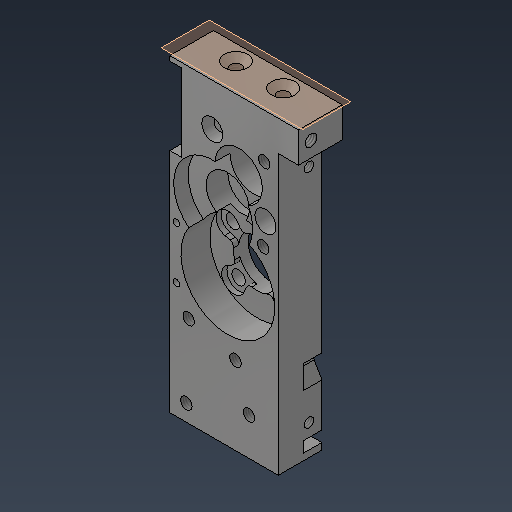
# Autodesk Inventor part: RightGearbox
Saved by Autodesk Inventor 2026.2 (Build 302298010, 298A)
## iProperties
Created: 2026-04-14
Part Number: RightGearbox
Material: Steel
Document SubType Name: Sheet Metal
Designer: szymo
Density: 7.85 g/cm^3
Appearance: Nylon 6(1)
Mass: 69.272 g
Surface Area: 68.2976 cm^2
Volume: 8.82446 cm^3
Sheet Metal Rule: Default
Author: szymo
Autodesk Inventor part; units mm, degrees
(part 1 of 2)
ref_plane "YZ Plane" through (0, 0, 0) normal (1, 0, 0) x (0, 1, 0)
ref_plane "XZ Plane" through (0, 0, 0) normal (0, 1, 0) x (-1, 0, 0)
ref_plane "XY Plane" through (0, 0, 0) normal (0, 0, 1) x (1, 0, 0)
sketch "Sketch1" plane through (0, 0, 0) normal (0, 0, 1) x (1, 0, 0)
  circle A0 centre (14.7, -14.7) radius 5
  circle A1 centre (14.7, -14.7) radius 14.7 construction
  circle A2 centre (14.7, -55.637072) radius 5
  circle A3 centre (14.7, -55.637072) radius 14.7 construction
  line L0 (23.1, 0) -> (0, 0)
  line L1 (0, 0) -> (0, -65.837072)
  line L2 (0, -65.837072) -> (23.1, -65.837072)
  line L3 (23.1, -65.837072) -> (23.1, 0)
  circle A4 centre (12.35, -35.272213) radius 5
  line L4 (23.43749, -53.479232) -> (27.439125, -51.168886)
  arc A5 (27.439125, -51.168886) -> (24.939125, -46.838759) centre (14.7, -55.637072) ccw
  line L5 (24.939125, -46.838759) -> (20.93749, -49.149105)
  arc A6 (23.43749, -53.479232) -> (20.93749, -49.149105) centre (14.7, -55.637072) ccw construction
  arc A7 (1.960875, -60.105258) -> (4.460875, -64.435385) centre (14.7, -55.637072) ccw
  line L6 (1.960875, -60.105258) -> (5.96251, -57.794913)
  line L7 (8.46251, -62.12504) -> (4.460875, -64.435385)
  line L8 (23.43749, -53.479232) -> (23.1, -53.479232)
  line L9 (24.939125, -46.838759) -> (23.1, -46.838759)
  line L10 (8.46251, -62.12504) -> (5.96251, -57.794913)
  line L11 (23.43749, -53.479232) -> (20.93749, -49.149105)
  line L12 (8.46251, -62.12504) -> (23.1, -62.12504)
  circle A8 centre (9.222618, -23.066498) radius 4.2 construction
  circle A9 centre (9.222618, -23.066498) radius 8 construction
  circle A10 centre (12.35, -35.272213) radius 9.6 construction
  circle A11 centre (12.35, -35.272213) radius 10
  circle A12 centre (9.222618, -23.066498) radius 4.6
  circle A13 centre (9.222618, -23.066498) radius 8.4
  arc A14 (5.96251, -57.794913) -> (8.46251, -62.12504) centre (14.7, -55.637072) ccw construction
  line L13 (2.5, -1) -> (1.5, -1)
  line L14 (1.5, -1) -> (1.5, -17)
  line L15 (1.5, -17) -> (2.5, -17)
  line L16 (2.5, -17) -> (2.5, -1)
  line L17 (1.5, -1) -> (1, -1)
  line L18 (1, -1) -> (1, -1)
  line L19 (1, -1) -> (0, -1)
  line L20 (2.5, -17) -> (2.5, -17.5)
  line L21 (2.5, -17.5) -> (1, -17.5)
  line L22 (1, -17.5) -> (1, -17.5)
  line L23 (1, -17.5) -> (0, -17.5)
  line L24 (23.1, 0) -> (27.4, 0)
  line L25 (27.4, 0) -> (27.4, -6.5)
  line L26 (27.4, -6.5) -> (23.1, -6.5)
  line L27 (24.939125, -23.498313) -> (20.93749, -21.187968)
  arc A15 (20.93749, -21.187968) -> (23.43749, -16.857841) centre (14.7, -14.7) ccw
  line L28 (23.43749, -16.857841) -> (27.439125, -19.168186)
  arc A16 (24.939125, -23.498313) -> (27.439125, -19.168186) centre (14.7, -14.7) ccw
  circle A17 centre (14.7, -14.7) radius 14.7 construction
  circle A18 centre (14.7, -14.7) radius 14 construction
  circle A19 centre (14.7, -14.7) radius 5
  circle A20 centre (14.7, -14.7) radius 14 construction
  line L29 (22.512272, -20.942468) -> (24.697093, -22.203875) construction
  arc A21 (22.512272, -20.942468) -> (24.012272, -18.344392) centre (14.7, -14.7) ccw construction
  line L30 (26.197093, -19.605799) -> (24.012272, -18.344392) construction
  arc A22 (24.697093, -22.203875) -> (26.197093, -19.605799) centre (14.7, -14.7) ccw construction
  circle A23 centre (14.7, -55.637072) radius 14.7 construction
  circle A24 centre (14.7, -55.637072) radius 14 construction
  line L31 (22.512272, -49.394604) -> (24.697093, -48.133197)
  arc A25 (26.197093, -50.731273) -> (24.697093, -48.133197) centre (14.7, -55.637072) ccw
  line L32 (26.197093, -50.731273) -> (24.012272, -51.99268)
  arc A26 (24.012272, -51.99268) -> (22.512272, -49.394604) centre (14.7, -55.637072) ccw
  arc A27 (3.202907, -60.542871) -> (4.702907, -63.140947) centre (14.7, -55.637072) ccw
  line L33 (3.202907, -60.542871) -> (5.387728, -59.281464)
  arc A28 (5.387728, -59.281464) -> (6.887728, -61.87954) centre (14.7, -55.637072) ccw
  line L34 (6.887728, -61.87954) -> (4.702907, -63.140947)
  circle A29 centre (14.7, -55.637072) radius 5
  circle A30 centre (14.7, -55.637072) radius 14 construction
  arc A31 (15.739868, -27.750823) -> (15.831115, -26.325602) centre (9.837244, -26.657388) ccw
  arc A32 (15.831115, -26.325602) -> (15.358114, -26.155676) centre (12.35, -35.272213) ccw
  arc A33 (15.358114, -26.155676) -> (14.521528, -27.313132) centre (19.770536, -30.225947) ccw
  arc A34 (14.521528, -27.313132) -> (14.102006, -27.210391) centre (12.35, -35.272213) ccw
  arc A35 (14.102006, -27.210391) -> (13.894939, -25.797343) centre (8.101031, -27.368074) ccw
  arc A36 (13.894939, -25.797343) -> (13.396945, -25.729472) centre (12.35, -35.272213) ccw
  arc A37 (13.396945, -25.729472) -> (12.819289, -27.035571) centre (18.559202, -28.793404) ccw
  arc A38 (12.819289, -27.035571) -> (12.387574, -27.022298) centre (12.35, -35.272213) ccw
  arc A39 (12.387574, -27.022298) -> (11.891242, -25.68318) centre (6.550518, -28.424209) ccw
  arc A40 (11.891242, -25.68318) -> (11.39002, -25.720331) centre (12.35, -35.272213) ccw
  arc A41 (11.39002, -25.720331) -> (11.09654, -27.117991) centre (17.076495, -27.644016) ccw
  arc A42 (11.09654, -27.117991) -> (10.671499, -27.194767) centre (12.35, -35.272213) ccw
  arc A43 (10.671499, -27.194767) -> (9.907595, -25.988105) centre (5.253471, -29.779634) ccw
  arc A44 (9.907595, -25.988105) -> (9.42505, -26.128654) centre (12.35, -35.272213) ccw
  arc A45 (9.42505, -26.128654) -> (9.428573, -27.556789) centre (15.387219, -26.828017) ccw
  arc A46 (9.428573, -27.556789) -> (9.028783, -27.720258) centre (12.35, -35.272213) ccw
  arc A47 (9.028783, -27.720258) -> (8.030693, -26.698789) centre (4.266575, -31.375112) ccw
  arc A48 (8.030693, -26.698789) -> (7.587914, -26.936594) centre (12.35, -35.272213) ccw
  arc A49 (7.587914, -26.936594) -> (7.888286, -28.332788) centre (13.565201, -26.381069) ccw
  arc A50 (7.888286, -28.332788) -> (7.53122, -28.575807) centre (12.35, -35.272213) ccw
  arc A51 (7.53122, -28.575807) -> (6.342565, -27.784174) centre (3.632965, -33.140911) ccw
  arc A52 (6.342565, -27.784174) -> (5.958905, -28.108841) centre (12.35, -35.272213) ccw
  arc A53 (5.958905, -28.108841) -> (6.542998, -29.412074) centre (11.690074, -26.322707) ccw
  arc A54 (6.542998, -29.412074) -> (6.24426, -29.72402) centre (12.35, -35.272213) ccw
  arc A55 (6.24426, -29.72402) -> (4.916991, -29.196821) centre (3.380331, -34.999859) ccw
  arc A56 (4.916991, -29.196821) -> (4.609216, -29.594161) centre (12.35, -35.272213) ccw
  arc A57 (4.609216, -29.594161) -> (5.451504, -30.747475) centre (9.843788, -26.655482) ccw
  arc A58 (5.451504, -30.747475) -> (5.224151, -31.114716) centre (12.35, -35.272213) ccw
  arc A59 (5.224151, -31.114716) -> (3.816275, -30.874993) centre (3.519714, -36.87071) ccw
  arc A60 (3.816275, -30.874993) -> (3.597838, -31.327639) centre (12.35, -35.272213) ccw
  arc A61 (3.597838, -31.327639) -> (4.661507, -32.28063) centre (8.107035, -27.364849) ccw
  arc A62 (4.661507, -32.28063) -> (4.515476, -32.687114) centre (12.35, -35.272213) ccw
  arc A63 (4.515476, -32.687114) -> (3.088524, -32.745344) centre (4.045023, -38.671698) ccw
  arc A64 (3.088524, -32.745344) -> (2.968971, -33.233515) centre (12.35, -35.272213) ccw
  arc A65 (2.968971, -33.233515) -> (4.207533, -33.944531) centre (6.555721, -28.419806) ccw
  arc A66 (4.207533, -33.944531) -> (4.149207, -34.372494) centre (12.35, -35.272213) ccw
  arc A67 (4.149207, -34.372494) -> (2.765544, -34.726131) centre (4.933299, -40.324113) ccw
  arc A68 (2.765544, -34.726131) -> (2.7501, -35.228491) centre (12.35, -35.272213) ccw
  arc A69 (2.7501, -35.228491) -> (4.109425, -35.666458) centre (5.257644, -29.774246) ccw
  arc A70 (4.109425, -35.666458) -> (4.141352, -36.097196) centre (12.35, -35.272213) ccw
  arc A71 (4.141352, -36.097196) -> (2.861451, -36.730784) centre (6.145721, -41.755736) ccw
  arc A72 (2.861451, -36.730784) -> (2.95079, -37.225378) centre (12.35, -35.272213) ccw
  arc A73 (2.95079, -37.225378) -> (4.37147, -37.371154) centre (4.269538, -31.368973) ccw
  arc A74 (4.37147, -37.371154) -> (4.492254, -37.785842) centre (12.35, -35.272213) ccw
  arc A75 (4.492254, -37.785842) -> (3.372052, -38.671691) centre (7.6293, -42.903997) ccw
  arc A76 (3.372052, -38.671691) -> (3.562271, -39.136902) centre (12.35, -35.272213) ccw
  arc A77 (3.562271, -39.136902) -> (4.982214, -38.984117) centre (3.634586, -33.134291) ccw
  arc A78 (4.982214, -38.984117) -> (5.186578, -39.36463) centre (12.35, -35.272213) ccw
  arc A79 (5.186578, -39.36463) -> (4.275033, -40.464025) centre (9.319196, -43.718713) ccw
  arc A80 (4.275033, -40.464025) -> (4.557818, -40.879521) centre (12.35, -35.272213) ccw
  arc A81 (4.557818, -40.879521) -> (5.914967, -40.434852) centre (3.38054, -34.993046) ccw
  arc A82 (5.914967, -40.434852) -> (6.193977, -40.76456) centre (12.35, -35.272213) ccw
  arc A83 (6.193977, -40.76456) -> (5.530929, -42.029451) centre (11.141552, -44.164277) ccw
  arc A84 (5.530929, -42.029451) -> (5.893921, -42.377073) centre (12.35, -35.272213) ccw
  arc A85 (5.893921, -42.377073) -> (7.128961, -41.659955) centre (3.518502, -36.864002) ccw
  arc A86 (7.128961, -41.659955) -> (7.470424, -41.924449) centre (12.35, -35.272213) ccw
  arc A87 (7.470424, -41.924449) -> (7.084851, -43.299554) centre (13.016724, -44.221214) ccw
  arc A88 (7.084851, -43.299554) -> (7.512186, -43.564109) centre (12.35, -35.272213) ccw
  arc A89 (7.512186, -43.564109) -> (8.571139, -42.605882) centre (4.042443, -38.665389) ccw
  arc A90 (8.571139, -42.605882) -> (8.960132, -42.793602) centre (12.35, -35.272213) ccw
  arc A91 (8.960132, -42.793602) -> (8.868885, -44.218823) centre (14.862756, -43.887037) ccw
  arc A92 (8.868885, -44.218823) -> (9.341886, -44.38875) centre (12.35, -35.272213) ccw
  arc A93 (9.341886, -44.38875) -> (10.178472, -43.231293) centre (4.929464, -40.318478) ccw
  arc A94 (10.178472, -43.231293) -> (10.597994, -43.334035) centre (12.35, -35.272213) ccw
  arc A95 (10.597994, -43.334035) -> (10.805061, -44.747083) centre (16.598969, -43.176351) ccw
  arc A96 (10.805061, -44.747083) -> (11.303055, -44.814954) centre (12.35, -35.272213) ccw
  arc A97 (11.303055, -44.814954) -> (11.880711, -43.508854) centre (6.140798, -41.751022) ccw
  arc A98 (11.880711, -43.508854) -> (12.312426, -43.522127) centre (12.35, -35.272213) ccw
  arc A99 (12.312426, -43.522127) -> (12.808758, -44.861245) centre (18.149482, -42.120216) ccw
  arc A100 (12.808758, -44.861245) -> (13.30998, -44.824094) centre (12.35, -35.272213) ccw
  arc A101 (13.30998, -44.824094) -> (13.60346, -43.426435) centre (7.623505, -42.90041) ccw
  arc A102 (13.60346, -43.426435) -> (14.028501, -43.349659) centre (12.35, -35.272213) ccw
  arc A103 (14.028501, -43.349659) -> (14.792405, -44.556321) centre (19.446529, -40.764791) ccw
  arc A104 (14.792405, -44.556321) -> (15.27495, -44.415771) centre (12.35, -35.272213) ccw
  arc A105 (15.27495, -44.415771) -> (15.271427, -42.987636) centre (9.312781, -43.716409) ccw
  arc A106 (15.271427, -42.987636) -> (15.671217, -42.824167) centre (12.35, -35.272213) ccw
  arc A107 (15.671217, -42.824167) -> (16.669307, -43.845636) centre (20.433425, -39.169314) ccw
  arc A108 (16.669307, -43.845636) -> (17.112086, -43.607831) centre (12.35, -35.272213) ccw
  arc A109 (17.112086, -43.607831) -> (16.811714, -42.211637) centre (11.134799, -44.163356) ccw
  arc A110 (16.811714, -42.211637) -> (17.16878, -41.968619) centre (12.35, -35.272213) ccw
  arc A111 (17.16878, -41.968619) -> (18.357435, -42.760252) centre (21.067035, -37.403514) ccw
  arc A112 (18.357435, -42.760252) -> (18.741095, -42.435585) centre (12.35, -35.272213) ccw
  arc A113 (18.741095, -42.435585) -> (18.157002, -41.132352) centre (13.009926, -44.221718) ccw
  arc A114 (18.157002, -41.132352) -> (18.45574, -40.820406) centre (12.35, -35.272213) ccw
  arc A115 (18.45574, -40.820406) -> (19.783009, -41.347604) centre (21.319669, -35.544567) ccw
  arc A116 (19.783009, -41.347604) -> (20.090784, -40.950264) centre (12.35, -35.272213) ccw
  arc A117 (20.090784, -40.950264) -> (19.248496, -39.79695) centre (14.856212, -43.888943) ccw
  arc A118 (19.248496, -39.79695) -> (19.475849, -39.42971) centre (12.35, -35.272213) ccw
  arc A119 (19.475849, -39.42971) -> (20.883725, -39.669433) centre (21.180286, -33.673716) ccw
  arc A120 (20.883725, -39.669433) -> (21.102162, -39.216786) centre (12.35, -35.272213) ccw
  arc A121 (21.102162, -39.216786) -> (20.038493, -38.263796) centre (16.592965, -43.179576) ccw
  arc A122 (20.038493, -38.263796) -> (20.184524, -37.857311) centre (12.35, -35.272213) ccw
  arc A123 (20.184524, -37.857311) -> (21.611476, -37.799082) centre (20.654977, -31.872727) ccw
  arc A124 (21.611476, -37.799082) -> (21.731029, -37.310911) centre (12.35, -35.272213) ccw
  arc A125 (21.731029, -37.310911) -> (20.492467, -36.599895) centre (18.144279, -42.12462) ccw
  arc A126 (20.492467, -36.599895) -> (20.550793, -36.171931) centre (12.35, -35.272213) ccw
  arc A127 (20.550793, -36.171931) -> (21.934456, -35.818295) centre (19.766701, -30.220312) ccw
  arc A128 (21.934456, -35.818295) -> (21.9499, -35.315935) centre (12.35, -35.272213) ccw
  arc A129 (21.9499, -35.315935) -> (20.590575, -34.877968) centre (19.442356, -40.77018) ccw
  arc A130 (20.590575, -34.877968) -> (20.558648, -34.44723) centre (12.35, -35.272213) ccw
  arc A131 (20.558648, -34.44723) -> (21.838549, -33.813641) centre (18.554279, -28.78869) ccw
  arc A132 (21.838549, -33.813641) -> (21.74921, -33.319048) centre (12.35, -35.272213) ccw
  arc A133 (21.74921, -33.319048) -> (20.32853, -33.173271) centre (20.430462, -39.175452) ccw
  arc A134 (20.32853, -33.173271) -> (20.207746, -32.758583) centre (12.35, -35.272213) ccw
  arc A135 (20.207746, -32.758583) -> (21.327948, -31.872734) centre (17.0707, -27.640428) ccw
  arc A136 (21.327948, -31.872734) -> (21.137729, -31.407523) centre (12.35, -35.272213) ccw
  arc A137 (21.137729, -31.407523) -> (19.717786, -31.560308) centre (21.065414, -37.410135) ccw
  arc A138 (19.717786, -31.560308) -> (19.513422, -31.179795) centre (12.35, -35.272213) ccw
  arc A139 (19.513422, -31.179795) -> (20.424967, -30.0804) centre (15.380804, -26.825712) ccw
  arc A140 (20.424967, -30.0804) -> (20.142182, -29.664905) centre (12.35, -35.272213) ccw
  arc A141 (20.142182, -29.664905) -> (18.785033, -30.109573) centre (21.31946, -35.551379) ccw
  arc A142 (18.785033, -30.109573) -> (18.506023, -29.779865) centre (12.35, -35.272213) ccw
  arc A143 (18.506023, -29.779865) -> (19.169071, -28.514974) centre (13.558448, -26.380149) ccw
  arc A144 (19.169071, -28.514974) -> (18.806079, -28.167352) centre (12.35, -35.272213) ccw
  arc A145 (18.806079, -28.167352) -> (17.571039, -28.884471) centre (21.181498, -33.680423) ccw
  arc A146 (17.571039, -28.884471) -> (17.229576, -28.619977) centre (12.35, -35.272213) ccw
  arc A147 (17.229576, -28.619977) -> (17.615149, -27.244871) centre (11.683276, -26.323211) ccw
  arc A148 (17.615149, -27.244871) -> (17.187814, -26.980316) centre (12.35, -35.272213) ccw
  arc A149 (17.187814, -26.980316) -> (16.128861, -27.938543) centre (20.657557, -31.879036) ccw
  arc A150 (16.128861, -27.938543) -> (15.739868, -27.750823) centre (12.35, -35.272213) ccw
  circle A151 centre (9.222618, -23.066498) radius 1.25
  arc A152 (17.179257, -22.234696) -> (16.013572, -21.994788) centre (15.595145, -26.979797) ccw
  arc A153 (16.013572, -21.994788) -> (15.948177, -21.640846) centre (9.222618, -23.066498) ccw
  arc A154 (15.948177, -21.640846) -> (16.951175, -21.000244) centre (13.776086, -17.134471) ccw
  arc A155 (16.951175, -21.000244) -> (16.832444, -20.598595) centre (9.222618, -23.066498) ccw
  arc A156 (16.832444, -20.598595) -> (15.642353, -20.606289) centre (16.269511, -25.569359) ccw
  arc A157 (15.642353, -20.606289) -> (15.504797, -20.273678) centre (9.222618, -23.066498) ccw
  arc A158 (15.504797, -20.273678) -> (16.352689, -19.43854) centre (12.443244, -16.31738) ccw
  arc A159 (16.352689, -19.43854) -> (16.153045, -19.070352) centre (9.222618, -23.066498) ccw
  arc A160 (16.153045, -19.070352) -> (14.99056, -19.325312) centre (16.635893, -24.049534) ccw
  arc A161 (14.99056, -19.325312) -> (14.786857, -19.028569) centre (9.222618, -23.066498) ccw
  arc A162 (14.786857, -19.028569) -> (15.442585, -18.035394) centre (10.969645, -15.795259) ccw
  arc A163 (15.442585, -18.035394) -> (15.170753, -17.716761) centre (9.222618, -23.066498) ccw
  arc A164 (15.170753, -17.716761) -> (14.08668, -18.207844) centre (16.67828, -22.486746) ccw
  arc A165 (14.08668, -18.207844) -> (13.825732, -17.959937) centre (9.222618, -23.066498) ccw
  arc A166 (13.825732, -17.959937) -> (14.260639, -16.852132) centre (9.419693, -15.590925) ccw
  arc A167 (14.260639, -16.852132) -> (13.928499, -16.596979) centre (9.222618, -23.066498) ccw
  arc A168 (13.928499, -16.596979) -> (12.970218, -17.302721) centre (16.394819, -20.949296) ccw
  arc A169 (12.970218, -17.302721) -> (12.663429, -17.114486) centre (9.222618, -23.066498) ccw
  arc A170 (12.663429, -17.114486) -> (12.858506, -15.940467) centre (7.861128, -15.71331) ccw
  arc A171 (12.858506, -15.940467) -> (12.480576, -15.759945) centre (9.222618, -23.066498) ccw
  arc A172 (12.480576, -15.759945) -> (11.689967, -16.649504) centre (15.797898, -19.504377) ccw
  arc A173 (11.689967, -16.649504) -> (11.350747, -16.529167) centre (9.222618, -23.066498) ccw
  arc A174 (11.350747, -16.529167) -> (11.297468, -15.340244) centre (6.362066, -16.157065) ccw
  arc A175 (11.297468, -15.340244) -> (10.890264, -15.242243) centre (9.222618, -23.066498) ccw
  arc A176 (10.890264, -15.242243) -> (10.301882, -16.27674) centre (14.913606, -18.21514) ccw
  arc A177 (10.301882, -16.27674) -> (9.945054, -16.22956) centre (9.222618, -23.066498) ccw
  arc A178 (9.945054, -16.22956) -> (9.64575, -15.077696) centre (4.988024, -16.902795) ccw
  arc A179 (9.64575, -15.077696) -> (9.227068, -15.066499) centre (9.222618, -23.066498) ccw
  arc A180 (9.227068, -15.066499) -> (8.866627, -16.200721) centre (13.78059, -17.137931) ccw
  arc A181 (8.866627, -16.200721) -> (8.507788, -16.228761) centre (9.222618, -23.066498) ccw
  arc A182 (8.507788, -16.228761) -> (7.975538, -15.164296) centre (3.799054, -17.917908) ccw
  arc A183 (7.975538, -15.164296) -> (7.563678, -15.240393) centre (9.222618, -23.066498) ccw
  arc A184 (7.563678, -15.240393) -> (7.446931, -16.424769) centre (12.448369, -16.319829) ccw
  arc A185 (7.446931, -16.424769) -> (7.101764, -16.526803) centre (9.222618, -23.066498) ccw
  arc A186 (7.101764, -16.526803) -> (6.359829, -15.596261) centre (2.84712, -19.158039) ccw
  arc A187 (6.359829, -15.596261) -> (5.972791, -15.756325) centre (9.222618, -23.066498) ccw
  arc A188 (5.972791, -15.756325) -> (6.104841, -16.939092) centre (10.975168, -15.796588) ccw
  arc A189 (6.104841, -16.939092) -> (5.78843, -17.110662) centre (9.222618, -23.066498) ccw
  arc A190 (5.78843, -17.110662) -> (4.869238, -16.35471) centre (2.173826, -20.568989) ccw
  arc A191 (4.869238, -16.35471) -> (4.523937, -16.591747) centre (9.222618, -23.066498) ccw
  arc A192 (4.523937, -16.591747) -> (4.899013, -17.721213) centre (9.425371, -15.591077) ccw
  arc A193 (4.899013, -17.721213) -> (4.625188, -17.954819) centre (9.222618, -23.066498) ccw
  arc A194 (4.625188, -17.954819) -> (3.568911, -17.406497) centre (1.808597, -22.089092) ccw
  arc A195 (3.568911, -17.406497) -> (3.280438, -17.710146) centre (9.222618, -23.066498) ccw
  arc A196 (3.280438, -17.710146) -> (3.882147, -18.736948) centre (7.866713, -15.712278) ccw
  arc A197 (3.882147, -18.736948) -> (3.662875, -19.022381) centre (9.222618, -23.066498) ccw
  arc A198 (3.662875, -19.022381) -> (2.515678, -18.705654) centre (1.767397, -23.651912) ccw
  arc A199 (2.515678, -18.705654) -> (2.296641, -19.062644) centre (9.222618, -23.066498) ccw
  arc A200 (2.296641, -19.062644) -> (3.098685, -19.941906) centre (6.367315, -16.154894) ccw
  arc A201 (3.098685, -19.941906) -> (2.943549, -20.26669) centre (9.222618, -23.066498) ccw
  arc A202 (2.943549, -20.26669) -> (1.75557, -20.1954) centre (2.052026, -25.189147) ccw
  arc A203 (1.75557, -20.1954) -> (1.615542, -20.59013) centre (9.222618, -23.066498) ccw
  arc A204 (1.615542, -20.59013) -> (2.582869, -21.283423) centre (4.992707, -16.89958) ccw
  arc A205 (2.582869, -21.283423) -> (2.498649, -21.633364) centre (9.222618, -23.066498) ccw
  arc A206 (2.498649, -21.633364) -> (1.321808, -21.810627) centre (2.650045, -26.633612) ccw
  arc A207 (1.321808, -21.810627) -> (1.266909, -22.225844) centre (9.222618, -23.066498) ccw
  arc A208 (1.266909, -22.225844) -> (2.357241, -22.702869) centre (3.802966, -17.91379) ccw
  arc A209 (2.357241, -22.702869) -> (2.347619, -23.062673) centre (9.222618, -23.066498) ccw
  arc A210 (2.347619, -23.062673) -> (1.23335, -23.480741) centre (3.535316, -27.922176) ccw
  arc A211 (1.23335, -23.480741) -> (1.265979, -23.898299) centre (9.222618, -23.066498) ccw
  arc A212 (1.265979, -23.898299) -> (2.431663, -24.138207) centre (2.85009, -19.153198) ccw
  arc A213 (2.431663, -24.138207) -> (2.497059, -24.492149) centre (9.222618, -23.066498) ccw
  arc A214 (2.497059, -24.492149) -> (1.49406, -25.132751) centre (4.669149, -28.998525) ccw
  arc A215 (1.49406, -25.132751) -> (1.612792, -25.534401) centre (9.222618, -23.066498) ccw
  arc A216 (1.612792, -25.534401) -> (2.802883, -25.526706) centre (2.175725, -20.563636) ccw
  arc A217 (2.802883, -25.526706) -> (2.940438, -25.859318) centre (9.222618, -23.066498) ccw
  arc A218 (2.940438, -25.859318) -> (2.092546, -26.694456) centre (6.001991, -29.815615) ccw
  arc A219 (2.092546, -26.694456) -> (2.29219, -27.062643) centre (9.222618, -23.066498) ccw
  arc A220 (2.29219, -27.062643) -> (3.454675, -26.807683) centre (1.809342, -22.083461) ccw
  arc A221 (3.454675, -26.807683) -> (3.658379, -27.104427) centre (9.222618, -23.066498) ccw
  arc A222 (3.658379, -27.104427) -> (3.00265, -28.097601) centre (7.47559, -30.337736) ccw
  arc A223 (3.00265, -28.097601) -> (3.274482, -28.416234) centre (9.222618, -23.066498) ccw
  arc A224 (3.274482, -28.416234) -> (4.358555, -27.925152) centre (1.766955, -23.646249) ccw
  arc A225 (4.358555, -27.925152) -> (4.619503, -28.173058) centre (9.222618, -23.066498) ccw
  arc A226 (4.619503, -28.173058) -> (4.184597, -29.280864) centre (9.025542, -30.54207) ccw
  arc A227 (4.184597, -29.280864) -> (4.516736, -29.536017) centre (9.222618, -23.066498) ccw
  arc A228 (4.516736, -29.536017) -> (5.475017, -28.830274) centre (2.050416, -25.1837) ccw
  arc A229 (5.475017, -28.830274) -> (5.781806, -29.018509) centre (9.222618, -23.066498) ccw
  arc A230 (5.781806, -29.018509) -> (5.586729, -30.192528) centre (10.584108, -30.419685) ccw
  arc A231 (5.586729, -30.192528) -> (5.964659, -30.37305) centre (9.222618, -23.066498) ccw
  arc A232 (5.964659, -30.37305) -> (6.755268, -29.483492) centre (2.647337, -26.628618) ccw
  arc A233 (6.755268, -29.483492) -> (7.094489, -29.603828) centre (9.222618, -23.066498) ccw
  arc A234 (7.094489, -29.603828) -> (7.147767, -30.792751) centre (12.08317, -29.97593) ccw
  arc A235 (7.147767, -30.792751) -> (7.554971, -30.890752) centre (9.222618, -23.066498) ccw
  arc A236 (7.554971, -30.890752) -> (8.143353, -29.856256) centre (3.531629, -27.917855) ccw
  arc A237 (8.143353, -29.856256) -> (8.500181, -29.903435) centre (9.222618, -23.066498) ccw
  arc A238 (8.500181, -29.903435) -> (8.799486, -31.0553) centre (13.457212, -29.230201) ccw
  arc A239 (8.799486, -31.0553) -> (9.218167, -31.066496) centre (9.222618, -23.066498) ccw
  arc A240 (9.218167, -31.066496) -> (9.578608, -29.932275) centre (4.664645, -28.995064) ccw
  arc A241 (9.578608, -29.932275) -> (9.937447, -29.904234) centre (9.222618, -23.066498) ccw
  arc A242 (9.937447, -29.904234) -> (10.469698, -30.968699) centre (14.646181, -28.215087) ccw
  arc A243 (10.469698, -30.968699) -> (10.881558, -30.892603) centre (9.222618, -23.066498) ccw
  arc A244 (10.881558, -30.892603) -> (10.998304, -29.708227) centre (5.996866, -29.813167) ccw
  arc A245 (10.998304, -29.708227) -> (11.343472, -29.606192) centre (9.222618, -23.066498) ccw
  arc A246 (11.343472, -29.606192) -> (12.085406, -30.536735) centre (15.598116, -26.974956) ccw
  arc A247 (12.085406, -30.536735) -> (12.472445, -30.37667) centre (9.222618, -23.066498) ccw
  arc A248 (12.472445, -30.37667) -> (12.340394, -29.193903) centre (7.470068, -30.336407) ccw
  arc A249 (12.340394, -29.193903) -> (12.656805, -29.022334) centre (9.222618, -23.066498) ccw
  arc A250 (12.656805, -29.022334) -> (13.575997, -29.778285) centre (16.27141, -25.564006) ccw
  arc A251 (13.575997, -29.778285) -> (13.921299, -29.541248) centre (9.222618, -23.066498) ccw
  arc A252 (13.921299, -29.541248) -> (13.546222, -28.411782) centre (9.019864, -30.541918) ccw
  arc A253 (13.546222, -28.411782) -> (13.820048, -28.178177) centre (9.222618, -23.066498) ccw
  arc A254 (13.820048, -28.178177) -> (14.876324, -28.726498) centre (16.636638, -24.043903) ccw
  arc A255 (14.876324, -28.726498) -> (15.164798, -28.422849) centre (9.222618, -23.066498) ccw
  arc A256 (15.164798, -28.422849) -> (14.563088, -27.396047) centre (10.578522, -30.420717) ccw
  arc A257 (14.563088, -27.396047) -> (14.782361, -27.110615) centre (9.222618, -23.066498) ccw
  arc A258 (14.782361, -27.110615) -> (15.929557, -27.427342) centre (16.677838, -22.481083) ccw
  arc A259 (15.929557, -27.427342) -> (16.148595, -27.070351) centre (9.222618, -23.066498) ccw
  arc A260 (16.148595, -27.070351) -> (15.34655, -26.19109) centre (12.077921, -29.978101) ccw
  arc A261 (15.34655, -26.19109) -> (15.501686, -25.866306) centre (9.222618, -23.066498) ccw
  arc A262 (15.501686, -25.866306) -> (16.689665, -25.937596) centre (16.393209, -20.943848) ccw
  arc A263 (16.689665, -25.937596) -> (16.829693, -25.542866) centre (9.222618, -23.066498) ccw
  arc A264 (16.829693, -25.542866) -> (15.862367, -24.849573) centre (13.452529, -29.233415) ccw
  arc A265 (15.862367, -24.849573) -> (15.946586, -24.499631) centre (9.222618, -23.066498) ccw
  arc A266 (15.946586, -24.499631) -> (17.123427, -24.322369) centre (15.795191, -19.499384) ccw
  arc A267 (17.123427, -24.322369) -> (17.178326, -23.907151) centre (9.222618, -23.066498) ccw
  arc A268 (17.178326, -23.907151) -> (16.087995, -23.430127) centre (14.642269, -28.219205) ccw
  arc A269 (16.087995, -23.430127) -> (16.097617, -23.070322) centre (9.222618, -23.066498) ccw
  arc A270 (16.097617, -23.070322) -> (17.211886, -22.652254) centre (14.90992, -18.210819) ccw
  arc A271 (17.211886, -22.652254) -> (17.179257, -22.234696) centre (9.222618, -23.066498) ccw
  circle A272 centre (9.222618, -23.066498) radius 1.25
  arc A273 (5.454719, -24.922014) -> (6.852049, -24.648554) centre (5.455154, -21.217462) ccw
  arc A274 (6.852049, -24.648554) -> (7.078829, -24.944441) centre (9.222618, -23.066498) ccw
  arc A275 (7.078829, -24.944441) -> (6.451609, -26.222684) centre (10.028976, -27.185053) ccw
  arc A276 (6.451609, -26.222684) -> (6.88728, -26.557371) centre (9.222618, -23.066498) ccw
  arc A277 (6.88728, -26.557371) -> (7.960673, -25.621883) centre (5.035381, -23.348917) ccw
  arc A278 (7.960673, -25.621883) -> (8.305014, -25.764738) centre (9.222618, -23.066498) ccw
  arc A279 (8.305014, -25.764738) -> (8.400947, -27.185339) centre (11.980222, -26.230092) ccw
  arc A280 (8.400947, -27.185339) -> (8.945593, -27.257352) centre (9.222618, -23.066498) ccw
  arc A281 (8.945593, -27.257352) -> (9.407435, -25.910499) centre (5.737574, -25.404699) ccw
  arc A282 (9.407435, -25.910499) -> (9.77707, -25.862045) centre (9.222618, -23.066498) ccw
  arc A283 (9.77707, -25.862045) -> (10.570451, -27.044355) centre (13.192571, -24.427448) ccw
  arc A284 (10.570451, -27.044355) -> (11.078134, -26.834396) centre (9.222618, -23.066498) ccw
  arc A285 (11.078134, -26.834396) -> (10.804674, -25.437067) centre (7.373582, -26.833961) ccw
  arc A286 (10.804674, -25.437067) -> (11.100561, -25.210286) centre (9.222618, -23.066498) ccw
  arc A287 (11.100561, -25.210286) -> (12.378804, -25.837506) centre (13.341173, -22.260139) ccw
  arc A288 (12.378804, -25.837506) -> (12.713491, -25.401835) centre (9.222618, -23.066498) ccw
  arc A289 (12.713491, -25.401835) -> (11.778003, -24.328442) centre (9.505037, -27.253735) ccw
  arc A290 (11.778003, -24.328442) -> (11.920859, -23.984101) centre (9.222618, -23.066498) ccw
  arc A291 (11.920859, -23.984101) -> (13.341459, -23.888168) centre (12.386212, -20.308893) ccw
  arc A292 (13.341459, -23.888168) -> (13.413472, -23.343522) centre (9.222618, -23.066498) ccw
  arc A293 (13.413472, -23.343522) -> (12.066619, -22.881681) centre (11.560819, -26.551541) ccw
  arc A294 (12.066619, -22.881681) -> (12.018165, -22.512045) centre (9.222618, -23.066498) ccw
  arc A295 (12.018165, -22.512045) -> (13.200475, -21.718665) centre (10.583568, -19.096545) ccw
  arc A296 (13.200475, -21.718665) -> (12.990516, -21.210981) centre (9.222618, -23.066498) ccw
  arc A297 (12.990516, -21.210981) -> (11.593187, -21.484441) centre (12.990081, -24.915534) ccw
  arc A298 (11.593187, -21.484441) -> (11.366406, -21.188554) centre (9.222618, -23.066498) ccw
  arc A299 (11.366406, -21.188554) -> (11.993626, -19.910311) centre (8.416259, -18.947942) ccw
  arc A300 (11.993626, -19.910311) -> (11.557955, -19.575624) centre (9.222618, -23.066498) ccw
  arc A301 (11.557955, -19.575624) -> (10.484562, -20.511112) centre (13.409855, -22.784078) ccw
  arc A302 (10.484562, -20.511112) -> (10.140221, -20.368257) centre (9.222618, -23.066498) ccw
  arc A303 (10.140221, -20.368257) -> (10.044288, -18.947656) centre (6.465013, -19.902903) ccw
  arc A304 (10.044288, -18.947656) -> (9.499642, -18.875644) centre (9.222618, -23.066498) ccw
  arc A305 (9.499642, -18.875644) -> (9.037801, -20.222496) centre (12.707661, -20.728297) ccw
  arc A306 (9.037801, -20.222496) -> (8.668165, -20.270951) centre (9.222618, -23.066498) ccw
  arc A307 (8.668165, -20.270951) -> (7.874785, -19.088641) centre (5.252665, -21.705547) ccw
  arc A308 (7.874785, -19.088641) -> (7.367101, -19.298599) centre (9.222618, -23.066498) ccw
  arc A309 (7.367101, -19.298599) -> (7.640561, -20.695929) centre (11.071654, -19.299034) ccw
  arc A310 (7.640561, -20.695929) -> (7.344674, -20.922709) centre (9.222618, -23.066498) ccw
  arc A311 (7.344674, -20.922709) -> (6.066432, -20.295489) centre (5.104062, -23.872856) ccw
  arc A312 (6.066432, -20.295489) -> (5.731744, -20.73116) centre (9.222618, -23.066498) ccw
  arc A313 (5.731744, -20.73116) -> (6.667232, -21.804553) centre (8.940198, -18.879261) ccw
  arc A314 (6.667232, -21.804553) -> (6.524377, -22.148894) centre (9.222618, -23.066498) ccw
  arc A315 (6.524377, -22.148894) -> (5.103776, -22.244827) centre (6.059023, -25.824102) ccw
  arc A316 (5.103776, -22.244827) -> (5.031764, -22.789473) centre (9.222618, -23.066498) ccw
  arc A317 (5.031764, -22.789473) -> (6.378617, -23.251315) centre (6.884417, -19.581454) ccw
  arc A318 (6.378617, -23.251315) -> (6.427071, -23.62095) centre (9.222618, -23.066498) ccw
  arc A319 (6.427071, -23.62095) -> (5.244761, -24.414331) centre (7.861667, -27.036451) ccw
  arc A320 (5.244761, -24.414331) -> (5.454719, -24.922014) centre (9.222618, -23.066498) ccw
  line L35 (1.5, -17) -> (1.5, -1)
  line L36 (2.5, -17) -> (1.5, -17)
  line L37 (2.5, -1) -> (2.5, -17)
  line L38 (2.5, -1) -> (1.5, -1)
  line L39 (4.460875, -64.435385) -> (23.1, -64.435385)
  point P0 (0, 0)
  point P1 (4.394176, -65.837072)
  point P2 (4.054242, -29.688272)
  point P3 (9.70004, -14.680076)
  point P4 (16.718073, -19.274645)
  point P5 (16.938443, -26.387046)
  point P6 (6.782075, -26.965696)
  point P7 (13.237489, -25.311672)
  point P8 (10.057406, -65.837072)
  point P9 (23.1, -47.900579)
  point P10 (23.1, -52.894682)
  dimension "d2" = 4.5
  dimension "d3" = 6.3
  dimension "d4" = 0.4
  dimension "d5" = 0.4
  dimension "d6" = 0.4
  dimension "d27" = 0
  dimension "d36" = 0.5
  dimension "d37" = 0
  dimension "d38" = 0.5
  dimension "d39" = 0.5
  dimension "d40" = 0
  dimension "d41" = 2
  dimension "d43" = 10
  dimension "d44" = 1
  dimension "d45" = 1
  dimension "d46" = 1
  dimension "d47" = 1
  dimension "d48" = 1
  dimension "d49" = 1
  dimension "d50" = 1
  dimension "d51" = 1
  dimension "d52" = 1
  dimension "d54" = 1
  dimension "d56" = 1
  dimension "d57" = 1
  dimension "d112" = 6.5
  constraints: 60 end point, 14 centre point, 13 coincident, 13 perpendicular, 12 point on circle, 7 parallel, 7 point on line, 6 tangent, 4 horizontal, 1 collinear, 1 vertical, 13 other
  measures "d2" distance edge to line of A3 L2
  measures "d3" distance edge to line of A1 L3
  measures "d27" distance from line of L6 A14.start
  measures "d36" distance between parallel lines of L14 L18
  measures "d37" distance between parallel lines of L19 L13
  measures "d38" distance between parallel lines of L22 L14
  measures "d39" distance between parallel lines of L21 L15
  measures "d40" distance between parallel lines of L21 L23
  measures "d41" distance edge to line of A1 L25
  measures "d43" diameter of A4
  measures "d44" distance between parallel lines of L28 L30
  measures "d45" distance between parallel lines of L27 L29
  measures "d46" radial gap between concentric circles of A22 A16
  measures "d47" radial gap between concentric circles of A15 A21
  measures "d48" distance between parallel lines of L32 L4
  measures "d49" distance between parallel lines of L5 L31
  measures "d50" radial gap between concentric circles of A5 A25
  measures "d51" radial gap between concentric circles of A6 A26
  measures "d52" radial gap between concentric circles of A28 A14
  measures "d54" radial gap between concentric circles of A7 A27
  measures "d56" distance between parallel lines of L6 L33
  measures "d57" distance between parallel lines of L7 L34
  measures "d112" distance between parallel lines of L26 L24
extrude "Extrusion5" add sketch "Sketch1" along normal blind 3.1 contours A0 A178 A179 A180 A181 A182 A183 A184 A185 A186 A187 A188 A189 A190 A191 A192 A193 A194 A195 A196 A197 A198 A199 A200 A201 A202 A203 A204 A205 A206 A207 A208 A209 A210 A211 A212 A213 A214 A215 A216 A217 A218 A219 A220 A221 A222 A223 A224 A225 A226 A227 A11 A13 | A13 A11 A262 A263 A264 A265 A266 A267 A268 A269 A270 A271 A152 A153 A154 A155 A156 A157 A158 A159 A0 | A0 A159 A158 A157 A156 A155 A154 A153 A152 A271 A270 A269 A268 A267 A266 A265 A264 A263 A262 A11 A12 A227 A226 A225 A224 A223 A222 A221 A220 A219 A218 A217 A216 A215 A214 A213 A212 A211 A210 A209 A208 A207 A206 A205 A204 A203 A202 A201 A200 A199 A198 A197 A196 A195 A194 A193 A192 A191 A190 A189 A188 A187 A186 A185 A184 A183 A182 A181 A180 A179 A178 | A13 A57 A58 A59 A60 A61 A62 A63 A64 A65 A66 A67 A68 A69 A70 A71 A72 A73 A74 A75 A76 A77 A78 A79 A80 A81 A82 A83 A84 A85 A86 A87 A88 A89 A90 A91 A92 A93 A94 A95 A96 A97 A98 A99 A100 A101 A102 A103 A104 A105 A106 A107 A108 A109 A110 A111 A112 A113 A114 A115 A116 A117 A118 A119 A120 A121 A122 A123 A124 A125 A126 A127 A128 A129 A130 A131 A132 A133 A134 A135 A136 A137 A138 A139 A140 A141 A142 A143 A144 A145 A146 A147 A148 A149 A150 A11 | A11 A227 A228 A56 A57 A13 | A11 A12 A49 A50 A51 A52 A53 A54 A55 A230 A229 A228 A56 A227 | A57 A56 A228 A55 A230 A231 A232 A233 A234 A235 A236 A237 A238 A239 A240 A241 A242 A4 A13 | A13 A4 A150 A149 A148 A147 A146 A145 A144 A143 A142 A141 A140 A139 A138 A137 A136 A135 A134 A133 A132 A131 A130 A129 A128 A127 A126 A125 A124 A123 A122 A121 A120 A119 A118 A117 A116 A115 A114 A113 A112 A111 A110 A109 A108 A107 A106 A105 A104 A103 A102 A101 A100 A99 A98 A97 A96 A95 A94 A93 A92 A91 A90 A89 A88 A87 A86 A85 A84 A83 A82 A81 A80 A79 A78 A77 A76 A75 A74 A73 A72 A71 A70 A69 A68 A67 A66 A65 A64 A63 A62 A61 A60 A59 A58 A57 | A13 A150 A31 A258 A259 A260 A32 A261 A262 A11 | A262 A261 A32 A33 A34 A35 A36 A37 A38 A39 A12 A11 | A13 A4 A248 A249 A250 A251 A252 A253 A254 A255 A256 A257 A258 A31 A150 | A12 A47 A46 A39 A38 A37 A36 A35 A34 A33 A32 A261 A260 A31 A258 A257 A256 A255 A254 A253 A252 A251 A250 A249 A248 A4 A246 A245 A244 A242 A241 A240 A239 A238 A237 A236 A235 A234 A233 A232 A231 A230 A55 A54 A53 A52 A51 A50 A49 | A56 A55 A228 | A12 A46 A47 | A228 A229 A230 A55 | A244 A245 A246 A4 | A32 A31 A260 A261 | A31 A260 A259 A258 | A2 | L3 A15 L27 L5 L11 L12 L10 L6 A7 L39 L2 L1 L23 L21 L20 L16 L13 L17 L19 L0 | L24 L25 L26 L3 | L3 L27 A15 | L3 L31 A26 L11 L5 | L39 L7 L12 L3 | L3 A26 L31 | A7 L6 L10 L7 | L33 A28 L34 A27
extrude "Extrusion6" add sketch "Sketch1" along normal blind 6.2 contours A0 A178 A179 A180 A181 A182 A183 A184 A185 A186 A187 A188 A189 A190 A191 A192 A193 A194 A195 A196 A197 A198 A199 A200 A201 A202 A203 A204 A205 A206 A207 A208 A209 A210 A211 A212 A213 A214 A215 A216 A217 A218 A219 A220 A221 A222 A223 A224 A225 A226 A227 A11 A13 | A13 A11 A262 A263 A264 A265 A266 A267 A268 A269 A270 A271 A152 A153 A154 A155 A156 A157 A158 A159 A0 | A0 A159 A158 A157 A156 A155 A154 A153 A152 A271 A270 A269 A268 A267 A266 A265 A264 A263 A262 A11 A12 A227 A226 A225 A224 A223 A222 A221 A220 A219 A218 A217 A216 A215 A214 A213 A212 A211 A210 A209 A208 A207 A206 A205 A204 A203 A202 A201 A200 A199 A198 A197 A196 A195 A194 A193 A192 A191 A190 A189 A188 A187 A186 A185 A184 A183 A182 A181 A180 A179 A178 | A2 | L3 A15 L27 L5 L11 L12 L10 L6 A7 L39 L2 L1 L23 L21 L20 L16 L13 L17 L19 L0 | L24 L25 L26 L3 | L3 L27 A15 | L3 L31 A26 L11 L5 | L39 L7 L12 L3 | L3 A26 L31 | A7 L6 L10 L7 | L33 A28 L34 A27
ref_plane "Work Plane3" through (6.764102, -40.858111, 9.3) normal (0, 0, 1) x (0.9993859, -0.0350396, 0)
extrude "Extrusion7" add sketch "Sketch1" along normal up to surface (9.3 mm away) contours A2 | L3 A15 L27 L5 L11 L12 L10 L6 A7 L39 L2 L1 L23 L21 L20 L16 L13 L17 L19 L0 | L24 L25 L26 L3 | L3 L27 A15 | L3 L31 A26 L11 L5 | L39 L7 L12 L3 | L3 A26 L31 | A7 L6 L10 L7 | L33 A28 L34 A27
extrude "Extrusion8" cut sketch "Sketch1" along normal blind 4 contours A2 | L3 L31 A26 L11 L5 | L39 L7 L12 L3 | L3 A26 L31 | A7 L6 L10 L7 | L33 A28 L34 A27
sketch "Sketch3" plane through (0, -65.837072, 9.3) normal (0, -1, 0) x (1, 0, 0)
  line L0 (23.1, -9.3) -> (23.1, 0) projected
  line L1 (23.1, 0) -> (0, 0) projected
  line L2 (0, -9.3) -> (0, 0) projected
  circle A0 centre (13.55, -3) radius 3
  circle A1 centre (7, -3) radius 3
  line L3 (4, -9.3) -> (4, 0)
  line L4 (0, -9.3) -> (23.1, -9.3) projected
  circle A2 centre (20.1, -3) radius 3
  line L5 (23.1, -9.3) -> (23.1, 0) projected
  line L6 (23.1, 0) -> (0, 0) projected
  point P0 (0, -9.3)
  dimension "d71" = 6
  dimension "d72" = 6
  dimension "d73" = 4
  dimension "d188" = 6
  dimension "d189" = 6.55
  dimension "d190" = 6.55
  constraints: 5 tangent, 3 centre point, 2 end point, 1 perpendicular, 1 point on line
  measures "d71" diameter of A1
  measures "d72" diameter of A0
  measures "d73" distance between parallel lines of L2 L3
  measures "d188" diameter of A2
  measures "d189" distance of A0.centre A2.centre
  measures "d190" distance of A1.centre A0.centre
hole "Hole1" at (13.55, -65.837072, 6.3) at (7, -65.837072, 6.3) at (20.1, -65.837072, 6.3) direction (0, 1, 0) diameter 2.459 depth 10 thread size "M3x0.5" class "6H" standard "ISO Metric profile"
sketch "Sketch4" plane through (0, 0, 9.3) normal (0, 0, 1) x (1, 0, 0)
  arc A0 (4.054242, -29.688272) -> (16.938443, -26.387046) centre (12.35, -35.272213) ccw
  arc A1 (9.70004, -14.680076) -> (4.054242, -29.688272) centre (9.222618, -23.066498) ccw
  arc A2 (16.718073, -19.274645) -> (9.70004, -14.680076) centre (14.7, -14.7) ccw
  arc A3 (16.938443, -26.387046) -> (16.718073, -19.274645) centre (9.222618, -23.066498) ccw
  line L0 (27.4, 0) -> (27.4, -6.5)
  line L1 (0, 0) -> (27.4, 0)
  line L2 (0, -1) -> (0, 0)
  line L3 (2.5, -1) -> (0, -1)
  line L4 (2.5, -17.5) -> (2.5, -1)
  line L5 (0, -17.5) -> (2.5, -17.5)
  line L6 (0, -65.837072) -> (0, -17.5)
  line L7 (23.1, -6.5) -> (23.1, -65.837072)
  line L8 (27.4, -6.5) -> (23.1, -6.5)
  line L9 (23.1, -6.5) -> (2.5, -6.5)
  line L10 (23.1, -19.5) -> (2.5, -19.5)
  circle A4 centre (16.825, -57.837072) radius 3
  circle A5 centre (3.5, -62.337072) radius 3.5
  line L11 (0, -65.837072) -> (0, 0)
  line L12 (23.1, -65.837072) -> (0, -65.837072)
  line L13 (23.1, -6.5) -> (23.1, -65.837072)
  circle A6 centre (20.104628, -9.5) radius 3
  circle A7 centre (20.104628, -9.5) radius 2.5
  arc A8 (16.718073, -19.274645) -> (9.70004, -14.680076) centre (14.7, -14.7) ccw
  circle A9 centre (4, -46.509539) radius 4
  circle A10 centre (14, -49.174641) radius 4
  arc A11 (4.054242, -29.688272) -> (16.938443, -26.387046) centre (12.35, -35.272213) ccw
  circle A12 centre (19.890727, -25.302888) radius 3
  circle A13 centre (19.890727, -25.302888) radius 2.5
  line L14 (23.1, -65.837072) -> (0, -65.837072)
  line L15 (21.3295, -65.837072) -> (18.8705, -65.837072)
  line L16 (14.7795, -65.837072) -> (12.3205, -65.837072)
  line L17 (12.3205, -55.837072) -> (14.7795, -55.837072)
  line L18 (21.3295, -65.837072) -> (18.8705, -65.837072)
  line L19 (18.8705, -55.837072) -> (21.3295, -55.837072)
  point P0 (0, -15)
  dimension "d85" = 6.5
  dimension "d86" = 19.5
  dimension "d87" = 6
  dimension "d88" = 7
  dimension "d89" = 6
  dimension "d90" = 5
  dimension "d92" = 8
  dimension "d93" = 8
  dimension "d94" = 6
  dimension "d95" = 5
  dimension "d103" = 10
  dimension "d191" = 5
  dimension "d192" = 4.5045
  dimension "d193" = 4.5045
  constraints: 9 tangent, 8 centre point, 4 end point, 4 point on line, 2 coincident, 1 parallel, 1 perpendicular
  measures "d85" distance between parallel lines of L1 L9
  measures "d86" distance between parallel lines of L1 L10
  measures "d87" diameter of A4
  measures "d88" diameter of A5
  measures "d89" diameter of A6
  measures "d90" diameter of A7
  measures "d92" diameter of A9
  measures "d93" diameter of A10
  measures "d94" diameter of A12
  measures "d95" diameter of A13
  measures "d103" horizontal distance of A9.centre A10.centre
  measures "d191" distance edge to line of A4 L12
  measures "d192" horizontal distance of A4.centre L19.end
  measures "d193" horizontal distance of A4.centre L17.start
sketch "Sketch12" plane through (0, 0, 9.3) normal (0, 0, 1) x (1, 0, 0)
  circle A0 centre (20.356854, -20.356854) radius 1.05643
  circle A1 centre (9.043146, -9.043146) radius 1.05643
  circle A2 centre (14.7, -14.7) radius 5
  circle A3 centre (14.7, -14.7) radius 14
  point P0 (0, 0)
hole "Hole9" at (9.043146, -9.043146, 9.3) at (20.356854, -20.356854, 9.3) direction (0, 0, -1) diameter 2.5 depth 10.3 counterbore diameter 4.5 counterbore depth 5.3
hole "Hole2" at (14, -49.174641, 9.3) at (19.890727, -25.302888, 9.3) at (16.825, -57.837072, 9.3) at (3.5, -62.337072, 9.3) at (4, -46.509539, 9.3) at (20.104628, -9.5, 9.3) direction (0, 0, -1) diameter 2.459 depth 15.55 thread size "M3x0.5" class "6H" standard "ISO Metric profile"
sketch "Sketch6" plane through (27.4, -6.5, 0) normal (1, 0, 0) x (0, 0, -1)
  line L0 (0, 0) -> (0, 6.5) projected
  line L1 (0, 6.5) -> (-9.3, 6.5) projected
  line L2 (-9.3, 6.5) -> (-9.3, 0) projected
  line L3 (0, 0) -> (-9.3, 0) projected
  line L4 (-4, 0) -> (-4, 6.5)
  line L5 (0, 0) -> (-9.3, 0) projected
  line L6 (-4, 0) -> (-9.3, 6.5)
  line L7 (-9.3, 6.5) -> (-9.3, 0) projected
  line L8 (-4, 6.5) -> (-9.3, 0)
  point P0 (0, 6.5)
  point P1 (-6.65, 3.25)
  dimension "d217" = 5.3
  constraints: 6 end point, 2 midpoint, 2 point on line, 1 perpendicular
  measures "d217" distance between parallel lines of L2 L4
hole "Hole4" at (27.4, -3.25, 6.65) direction (-1, 0, 0) diameter 2.459 depth 10 thread size "M3x0.5" class "6H" standard "ISO Metric profile"
sketch "Sketch5" plane through (0, -65.837072, 0) normal (-1, 0, 0) x (0, 0, 1)
  line L0 (0, 40.042024) -> (0, 20.295048)
  line L1 (0, 40.042024) -> (-3.8, 40.042024)
  circle A0 centre (-1.9, 30.668536) radius 1.0065
  line L2 (0, 20.295048) -> (-3.8, 20.295048)
  line L3 (-3.8, 40.042024) -> (-3.8, 20.295048)
  point P0 (0, 65.837072)
hole "Hole3" at (0, -35.168536, -1.9) direction (1, 0, 0) diameter 2.9 end through all countersink diameter 7 countersink angle 90 clearance for "Countersunk Flat Head Screw ISO 2009/7046" size "M2.5" standard "ISO"
sketch "Sketch7" plane through (23.1, -65.837072, 9.3) normal (1, 0, 0) x (0, 0, -1)
  line L0 (5.3, 1.401687) -> (5.3, 3.712032)
  line L1 (9.3, 59.337072) -> (0, 59.337072)
  line L2 (0, 59.337072) -> (0, 0)
  line L3 (9.3, 0) -> (0, 0)
  circle A0 centre (6.55, 53.607572) radius 2.75
  line L4 (9.3, 59.337072) -> (0, 59.337072)
  circle A1 centre (6.55, 6.462032) radius 2.75
  line L5 (5.3, 17.936494) -> (9.3, 17.936494)
  line L6 (9.3, 17.936494) -> (9.3, 59.337072)
  line L7 (9.3, 0) -> (9.3, 1.401687)
  line L8 (9.3, 12.94239) -> (5.3, 12.94239)
  line L9 (9.3, 1.401687) -> (5.3, 1.401687)
  line L10 (5.3, 3.712032) -> (9.3, 3.712032)
  line L11 (9.3, 3.712032) -> (9.3, 12.94239)
  line L12 (5.3, 12.94239) -> (5.3, 17.936494)
  line L13 (9.3, 57.566572) -> (9.3, 55.107572)
  line L14 (0, 55.107572) -> (0, 57.566572)
  point P0 (9.3, 65.837072)
  dimension "d122" = 5.5
  dimension "d123" = 5.5
  dimension "d194" = 1.5
  constraints: 3 tangent, 2 centre point
  measures "d122" diameter of A0
  measures "d123" diameter of A1
  measures "d194" vertical distance of A0.centre L13.end
hole "Hole5" at (23.1, -59.37504, 2.75) at (23.1, -12.2295, 2.75) direction (-1, 0, 0) diameter 2.013 depth 8 thread size "M2.5x0.45" class "6H" standard "ISO Metric profile"